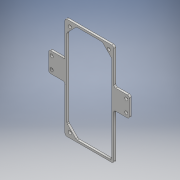
# Autodesk Inventor part: PCB Holder
Saved by Autodesk Inventor 2017 (Build 210142000, 142)
## iProperties
Created: 2017-05-28
Part Number: PCB Holder
Material: Generic
Document SubType Name: Modeling
Designer: William
Density: 1 g/cm^3
Appearance: Default
Author: William
Autodesk Inventor part; units mm, degrees
ref_plane "YZ Plane" through (0, 0, 0) normal (1, 0, 0) x (0, 1, 0)
ref_plane "XZ Plane" through (0, 0, 0) normal (0, 1, 0) x (-1, 0, 0)
ref_plane "XY Plane" through (0, 0, 0) normal (0, 0, 1) x (1, 0, 0)
sketch "Sketch1" plane through (0, 0, 0) normal (0, 1, 0) x (-1, 0, 0)
  line L0 (-0.3716, 0) -> (46.6284, 0) construction
  line L1 (46.6284, 0) -> (46.6284, -99) construction
  line L2 (46.6284, -100) -> (-0.3716, -100) construction
  line L3 (-0.3716, -100) -> (-0.3716, -1) construction
  circle A0 centre (3.6284, -4) radius 1.6 construction
  circle A1 centre (42.6284, -4) radius 1.6 construction
  circle A2 centre (42.6284, -96) radius 1.729 construction
  line L4 (23.1284, 0) -> (23.1284, -100) construction
  line L5 (23.1284, -13) -> (18.1284, -13) construction
  line L6 (18.1284, -13) -> (0.1284, -13) construction
  line L7 (23.1284, -13) -> (46.1284, -13) construction
  line L8 (45.6284, -10.5) -> (45.6284, -89.5)
  line L9 (10.1284, -1) -> (36.1284, -1)
  line L10 (0.6284, -99) -> (36.1284, -99)
  line L11 (0.6284, -10.5) -> (0.6284, -99)
  line L12 (36.9206, -1) -> (49.2353, -1) construction
  line L13 (45.6284, -1) -> (36.1284, -1) construction
  line L14 (36.1284, -1) -> (45.6284, -10.5)
  line L15 (36.1284, -99) -> (45.6284, -89.5)
  line L16 (36.1284, -99) -> (49.5635, -99) construction
  line L17 (0.6284, -1) -> (10.1284, -1) construction
  line L18 (10.1284, -1) -> (0.6284, -10.5)
  circle A3 centre (3.6284, -4) radius 1.6
  circle A4 centre (42.6284, -4) radius 1.6
  circle A5 centre (42.6284, -96) radius 1.729
  circle A6 centre (61, -38.5) radius 1.6
  circle A7 centre (61, -50.5) radius 1.6
  line L19 (47.6284, -34.5) -> (64, -34.5)
  line L20 (64, -34.5) -> (64, -54.5)
  line L21 (64, -54.5) -> (47.6284, -54.5)
  circle A8 centre (-14, -38.5) radius 1.6
  circle A9 centre (-14, -50.5) radius 1.6
  line L22 (-1.3716, -34.5) -> (-17, -34.5)
  line L23 (-17, -34.5) -> (-17, -54.5)
  line L24 (-17, -54.5) -> (-1.3716, -54.5)
  line L25 (47.6284, -101) -> (47.6284, -54.5)
  line L26 (47.6284, -34.5) -> (47.6284, 1)
  line L27 (-1.3716, -101) -> (-1.3716, -54.5)
  line L28 (-1.3716, -34.5) -> (-1.3716, 1)
  line L29 (47.6284, 1) -> (-1.3716, 1)
  line L30 (47.6284, -101) -> (-1.3716, -101)
  dimension "d0" = 47
  dimension "d1" = 100
  dimension "d2" = 3.2
  dimension "d3" = 4
  dimension "d4" = 4
  dimension "d5" = 4
  dimension "d6" = 43
  dimension "d7" = 3.2
  dimension "d8" = 43
  dimension "d9" = 96
  dimension "d10" = 23.5
  dimension "d11" = 5
  dimension "d12" = 13
  dimension "d13" = 18
  dimension "d15" = 23
  dimension "d24" = 1
  dimension "d33" = 8.7079
  dimension "d34" = 9.5
  dimension "d35" = 45
  dimension "d36" = 45
  dimension "d37" = 9.5
  dimension "d38" = 45
  dimension "d39" = 3.2
  dimension "d42" = 3.2
  dimension "d43" = 12
  dimension "d44" = 4
  dimension "d45" = 3
  dimension "d46" = 4
  dimension "d47" = 3.2
  dimension "d49" = 3.2
  dimension "d50" = 12
  dimension "d51" = 3
  constraints: 62 end point, 10 centre point, 8 horizontal, 8 parallel, 5 perpendicular, 4 point on line, 3 coincident, 3 concentric, 2 midpoint, 1 equal length
  measures "d0" distance of L2.start L3.start
  measures "d1" distance of L0.end L2.start
  measures "d2" diameter of A0
  measures "d3" distance from line of L0 A0.centre
  measures "d4" distance from line of L3 A0.centre
  measures "d5" distance from line of L0 A1.centre
  measures "d6" distance from line of L3 A1.centre
  measures "d7" diameter of A1
  measures "d8" distance from line of L3 A2.centre
  measures "d9" distance from line of L0 A2.centre
  measures "d10" distance between parallel lines of L3 L4
  measures "d11" distance of L7.start L6.start
  measures "d12" distance between parallel lines of L0 L5
  measures "d13" distance of L6.start L6.end
  measures "d15" distance of L7.start L7.end
  measures "d24" distance between parallel lines of L8 L1
  measures "d33" distance of L13.start L12.start
  measures "d34" distance of L9.end L13.start
  measures "d35" angle of L14 L12
  measures "d36" angle of L16 L15
  measures "d37" distance of L9.start L17.start
  measures "d38" angle of L17 L18
  measures "d39" diameter of A6
  measures "d42" diameter of A7
  measures "d43" distance of A6.centre A7.centre
  measures "d44" distance from line of A6.centre L19
  measures "d45" distance from line of L20 A6.centre
  measures "d46" distance from line of L21 A7.centre
  measures "d47" diameter of A8
  measures "d49" diameter of A9
  measures "d50" distance of A9.centre A8.centre
  measures "d51" distance from line of L23 A8.centre
extrude "Extrusion1" add sketch "Sketch1" along normal blind 2
fillet "Fillet1" radius 2 18 edges at (-45.6284, 1, -89.5) (-36.1284, 1, -99) (-64, 1, -34.5) (-47.6284, 1, 1) (1.3716, 1, 1) (17, 1, -34.5) (1.3716, 1, -34.5) (17, 1, -54.5) (1.3716, 1, -54.5) (1.3716, 1, -101) (-47.6284, 1, -101) (-64, 1, -54.5) (-45.6284, 1, -10.5) (-36.1284, 1, -1) (-10.1284, 1, -1) (-0.6284, 1, -10.5) (-47.6284, 1, -54.5) (-0.6284, 1, -99)
body "Solid1"
